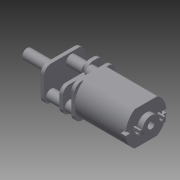
# Autodesk Inventor part: Motor
Saved by Autodesk Inventor 2015 (Build 190159000, 159)
## iProperties
Created: 2019-01-15
Part Number: Motor
Material: Типовые
Document SubType Name: Modeling
Designer: kostya
Density: 1 g/cm^3
Appearance: По умолчанию
Author: kostya
Autodesk Inventor part; units mm, degrees
ref_plane "YZ Plane" through (0, 0, 0) normal (1, 0, 0) x (0, 1, 0)
sketch "Эскиз1" plane through (0, 0, 0) normal (0, 0, 1) x (1, 0, 0)
  line L0 (-4.5, -6) -> (4.5, -6)
  line L1 (4.5, -6) -> (4.5, 6)
  line L2 (4.5, 6) -> (-4.5, 6)
  line L3 (-4.5, 6) -> (-4.5, -6)
  line L4 (-4.5, -6) -> (4.5, 6) construction
  line L5 (4.5, -6) -> (-4.5, 6) construction
  point P0 (0, 0)
  dimension "d0" = 9
  dimension "d1" = 12
  constraints: 12 end point, 2 midpoint, 2 parallel, 1 horizontal, 1 perpendicular
  measures "d0" distance of L2.end L1.end
  measures "d1" distance of L1.end L0.end
extrude "Выдавливание1" add sketch "Эскиз1" against normal blind 10
sketch "Эскиз2" plane through (4.5, -6, 0) normal (1, 0, 0) x (0, 0, -1)
  line L0 (0, 0) -> (0, 12) projected
  line L1 (0, 0) -> (10, 0) projected
  line L2 (10, 12) -> (10, 0) projected
  line L3 (0, 12) -> (10, 12) projected
  line L4 (0, 12) -> (10, 12) construction
  line L5 (5, 12) -> (5, 0) construction
  line L6 (10, 0) -> (10, 12) construction
  line L7 (10, 6) -> (0, 6) construction
  arc A0 (10, 9.3166) -> (0, 9.3166) centre (5, 6) ccw
  arc A1 (0, 2.6834) -> (10, 2.6834) centre (5, 6) ccw
  line L8 (0, 9.3166) -> (0, 2.6834)
  line L9 (0, 12) -> (0, 0) projected
  line L10 (10, 9.3166) -> (10, 2.6834)
  constraints: 8 end point, 5 point on circle, 4 midpoint, 4 point on line, 2 centre point, 1 collinear, 1 horizontal, 1 parallel
extrude "Выдавливание2" add sketch "Эскиз2" along normal blind 15 contours L0 A0 L2 A1
sketch "Эскиз3" plane through (19.5, -6, 0) normal (1, 0, 0) x (0, 0, -1)
  line L0 (0, 9.3166) -> (0, 2.6834) projected
  arc A0 (0, 2.6834) -> (10, 2.6834) centre (5, 6) ccw projected
  line L1 (10, 2.6834) -> (10, 9.3166) projected
  arc A1 (10, 9.3166) -> (0, 9.3166) centre (5, 6) ccw projected
  circle A2 centre (5, 6) radius 2.5
  circle A3 centre (5, 6) radius 1
  line L2 (5, 8.5) -> (5, 9.5) construction
  line L3 (4.25, 9.75) -> (5.75, 9.75)
  line L4 (5.75, 9.75) -> (5.75, 9.25)
  line L5 (5.75, 9.25) -> (4.25, 9.25)
  line L6 (4.25, 9.25) -> (4.25, 9.75)
  line L7 (4.25, 9.75) -> (5.75, 9.25) construction
  line L8 (5.75, 9.75) -> (4.25, 9.25) construction
  line L9 (10, 2.6834) -> (10, 9.3166) construction
  line L10 (10, 6) -> (0, 6) construction
  line L11 (4.25, 2.25) -> (5.75, 2.25)
  line L12 (5.75, 2.25) -> (5.75, 2.75)
  line L13 (5.75, 2.75) -> (4.25, 2.75)
  line L14 (4.25, 2.75) -> (4.25, 2.25)
  dimension "d6" = 5
  dimension "d7" = 2
  dimension "d9" = 1
  dimension "d10" = 1.5
  dimension "d11" = 0.5
  constraints: 24 end point, 4 symmetric about line, 3 midpoint, 2 coincident, 2 parallel, 2 perpendicular, 1 centre point, 1 horizontal, 1 vertical, 1 vertical alignment, 2 other
  measures "d7" diameter of A3
  measures "d9" distance of L2.start L2.end
  measures "d10" distance of L3.start L3.end
  measures "d11" distance of L3.end L4.end
extrude "Выдавливание3" add sketch "Эскиз3" along normal blind 1.5 contours A2
extrude "Выдавливание4" add sketch "Эскиз3" along normal blind 2 contours L3 L4 L5 L6 | L14 L13 L12 L11
sketch "Эскиз4" plane through (19.5, 3.75, -4.25) normal (0, 1, 0) x (1, 0, 0)
  line L0 (0, 0) -> (0, 1.5) projected
  line L1 (0, 0) -> (2, 0) projected
  line L2 (2, 1.5) -> (2, 0) projected
  line L3 (0, 1.5) -> (2, 1.5) projected
  circle A0 centre (1, 0.75) radius 0.65
  point P0 (-19.5, -4.25)
  dimension "d16" = 1.3
  constraints: 1 centre point
  measures "d16" diameter of A0
extrude "Выдавливание5" cut sketch "Эскиз4" against normal blind 1 contours A0
ref_plane "РабПлоскость1" through (19.5, 0, -4.25) normal (0, 1, 0) x (1, 0, 0)
mirror "Зеркальное отражение1" about plane through (19.5, 0, -4.25) normal (0, 1, 0) of "Выдавливание5"
sketch "Эскиз5" plane through (19.5, -6, 0) normal (1, 0, 0) x (0, 0, -1)
  line L0 (5.75, 9.75) -> (5.75, 9.25) projected
  line L1 (5.75, 9.25) -> (4.25, 9.25) projected
  line L2 (4.25, 9.25) -> (4.25, 9.75) projected
  line L3 (4.25, 9.75) -> (5.75, 9.75) projected
  line L4 (4.25, 2.25) -> (4.25, 2.75) projected
  line L5 (4.25, 2.75) -> (5.75, 2.75) projected
  line L6 (5.75, 2.75) -> (5.75, 2.25) projected
  line L7 (5.75, 2.25) -> (4.25, 2.25) projected
  line L8 (0, 9.3166) -> (0, 2.6834) projected
  arc A0 (0, 2.6834) -> (10, 2.6834) centre (5, 6) ccw projected
  line L9 (10, 2.6834) -> (10, 9.3166) projected
  arc A1 (10, 9.3166) -> (0, 9.3166) centre (5, 6) ccw projected
  circle A2 centre (5, 6) radius 2.5 projected
  line L10 (5, 2.25) -> (5, 1.25) construction
  line L11 (5.5, 1.25) -> (5, 1.25) construction
  line L12 (5, 1.25) -> (4.5, 1.25) construction
  line L13 (4.5, 1.25) -> (5.5, 1.25)
  line L14 (5.5, 1.25) -> (5.5, -0.0734)
  line L15 (5.5, -0.0734) -> (4.5, -0.0734)
  line L16 (4.5, -0.0734) -> (4.5, 1.25)
  line L17 (5, 6) -> (10, 6) construction
  line L18 (10, 2.6834) -> (10, 9.3166) construction
  line L19 (5, 9.75) -> (5, 10.75) construction
  line L20 (5.5, 10.75) -> (5, 10.75) construction
  line L21 (4.5, 10.75) -> (5.5, 10.75)
  line L22 (5.5, 10.75) -> (5.5, 12.0734)
  line L23 (5.5, 12.0734) -> (4.5, 12.0734)
  line L24 (4.5, 12.0734) -> (4.5, 10.75)
  point P0 (0, 6)
  dimension "d19" = 1
  dimension "d20" = 0.5
  constraints: 28 end point, 7 symmetric about line, 2 horizontal, 2 midpoint, 2 parallel, 2 point on line, 1 perpendicular, 1 vertical
  measures "d19" distance of L10.start L10.end
  measures "d20" distance of L10.end L12.end
extrude "Выдавливание6" cut sketch "Эскиз5" against normal blind 1.5 contours L24 L23 L22 A1 | A1 L22 L21 L24 | L16 L13 L14 A0 | A0 L14 L15 L16
sketch "Эскиз6" plane through (-4.5, -6, 0) normal (0, -1, 0) x (1, 0, 0)
  line L0 (0, 0) -> (9, 0) projected
  line L1 (0, 0) -> (0, -10) projected
  line L2 (9, -10) -> (0, -10) projected
  line L3 (9, -5) -> (9, -10) projected
  line L4 (9, 0) -> (9, -5) projected
  line L5 (9, 0) -> (8, 0)
  line L6 (8, 0) -> (8, -10)
  line L7 (8, -10) -> (9, -10)
  line L8 (9, -10) -> (9, 0)
  point P0 (4.5, 0)
  dimension "d23" = 1
  constraints: 8 end point, 2 parallel, 1 horizontal, 1 perpendicular, 1 point on line
  measures "d23" distance of L7.end L6.end
extrude "Выдавливание7" cut sketch "Эскиз6" against normal up to next contours L0 L6 L2 L1
sketch "Эскиз7" plane through (3.5, -6, -10) normal (-1, 0, 0) x (0, 0, 1)
  line L0 (0, 12) -> (10, 12) projected
  line L1 (0, 0) -> (0, 12) projected
  line L2 (10, 0) -> (0, 0) projected
  line L3 (10, 12) -> (10, 0) projected
  line L4 (0, 0) -> (1, 0) construction
  line L5 (1, 0) -> (1, 1) construction
  line L6 (1, 1) -> (0, 1) construction
  line L7 (0, 1) -> (0, 0) construction
  line L8 (1, 1) -> (3.1213, 3.1213) construction
  line L9 (1, 1) -> (4, 1) construction
  circle A0 centre (2.0607, 2.0607) radius 1.5
  point P0 (10, 6)
  dimension "d26" = 1
  dimension "d27" = 1
  dimension "d28" = 3
  dimension "d29" = 45
  constraints: 12 end point, 2 horizontal, 2 parallel, 1 equal length, 1 midpoint, 1 perpendicular, 3 other
  measures "d26" distance of L6.end L5.end
  measures "d27" distance of L5.end L4.end
  measures "d28" distance of L5.end L8.end
  measures "d29" angle of L9 L8
extrude "Выдавливание8" add sketch "Эскиз7" along normal blind 2.5 contours A0
sketch "Эскиз8" plane through (4.5, -6, -10) normal (0, -1, 0) x (1, 0, 0)
  line L0 (-3.5, 3.5607) -> (-3.5, 0.5607) projected
  line L1 (-1, 0.5607) -> (-1, 3.5607) projected
  line L2 (-1, 10) -> (-1, 0) construction
  line L3 (0, 0) -> (-1, 0) construction
  line L4 (0, 5) -> (0, 0) construction
  line L5 (0, 10) -> (0, 5) construction
  line L6 (-1, 10) -> (0, 10) construction
  line L7 (0, 0) -> (-4.7525, 0) construction
  line L8 (-3.5, 0.5607) -> (-3.5, 0) construction
  line L9 (-3.5, 0) -> (-4.5, 0)
  line L10 (-4.5, 0) -> (-4.5, 10)
  line L11 (-4.5, 10) -> (-3.5, 10)
  line L12 (-3.5, 10) -> (-3.5, 0)
  dimension "d32" = 1
  constraints: 12 end point, 2 horizontal, 2 parallel, 2 perpendicular, 1 point on line
  measures "d32" distance of L10.end L11.end
extrude "Выдавливание9" add sketch "Эскиз8" against normal up to surface (12 mm away)
sketch "Эскиз9" plane through (0, -6, -10) normal (-1, 0, 0) x (0, 0, 1)
  line L0 (10, 12) -> (0, 12) projected
  line L1 (0, 0) -> (0, 12) projected
  line L2 (10, 0) -> (0, 0) projected
  line L3 (10, 0) -> (10, 12) projected
  line L4 (10, 12) -> (10, 7) construction
  line L5 (10, 12) -> (10, 0) construction
  line L6 (0, 0) -> (7.5, 0) construction
  line L7 (10, 0) -> (0, 0) construction
  line L8 (10, 7) -> (7.5, 7)
  line L9 (7.5, 7) -> (7.5, 0)
  line L10 (7.5, 0) -> (10, 0)
  line L11 (10, 0) -> (10, 7)
  point P0 (10, 6)
  dimension "d35" = 5
  dimension "d36" = 7.5
  constraints: 12 end point, 2 parallel, 2 point on line, 1 horizontal, 1 perpendicular
  measures "d35" distance of L0.start L4.end
  measures "d36" distance of L1.start L6.end
extrude "Выдавливание10" cut sketch "Эскиз9" against normal blind 2.5 contours L3 L2 L9 L8
sketch "Эскиз10" plane through (0, -6, -10) normal (-1, 0, 0) x (0, 0, 1)
  line L0 (7.5, 7) -> (10, 7) projected
  line L1 (10, 7) -> (10, 12) projected
  line L2 (10, 12) -> (0, 12) projected
  line L3 (0, 0) -> (0, 12) projected
  line L4 (7.5, 0) -> (0, 0) projected
  line L5 (7.5, 0) -> (7.5, 7) projected
  circle A0 centre (2.0607, 2.0607) radius 1.5 projected
  point P0 (10, 6)
extrude "Выдавливание11" add sketch "Эскиз10" along normal blind 4.5 contours A0
sketch "Эскиз11" plane through (4.5, -6, -10) normal (0, -1, 0) x (1, 0, 0)
  line L0 (-3.5, 7.5) -> (-4.5, 7.5) projected
  line L1 (-4.5, 7.5) -> (-4.5, 0) projected
  line L2 (-4.5, 0) -> (-3.5, 0) projected
  line L3 (-3.5, 0) -> (-3.5, 7.5) projected
  line L4 (-3.5, 10) -> (-3.5, 7.5) projected
  line L5 (-4.5, 10) -> (-3.5, 10) projected
  line L6 (-4.5, 7.5) -> (-4.5, 10) projected
  line L7 (-4.5, 7.5) -> (-3.5, 7.5) projected
  line L8 (-1, 10) -> (-1, 0) projected
  line L9 (0, 0) -> (-1, 0) projected
  line L10 (0, 5) -> (0, 0) projected
  line L11 (0, 10) -> (0, 5) projected
  line L12 (-1, 10) -> (0, 10) projected
  line L13 (-9, 3.5607) -> (-9, 0.5607) projected
  line L14 (-4.5, 0.5607) -> (-4.5, 3.5607) projected
  line L15 (-9, 0.5607) -> (-9, 0) construction
  line L16 (-9, 0) -> (0, 0) construction
  line L17 (-9, 0) -> (-10, 0)
  line L18 (-10, 0) -> (-10, 10)
  line L19 (-10, 10) -> (-9, 10)
  line L20 (-9, 10) -> (-9, 0)
  dimension "d41" = 1
  constraints: 12 end point, 2 parallel, 2 perpendicular, 1 horizontal, 1 vertical
  measures "d41" distance of L18.end L19.end
extrude "Выдавливание12" add sketch "Эскиз11" against normal up to surface (12 mm away) contours L13 L20 L17 L18 L19
ref_plane "РабПлоскость3" through (4.5, -6, 0) normal (0, -0.7071068, -0.7071068) x (1, 0, 0)
mirror "Зеркальное отражение2" about plane through (4.5, -6, 0) normal (0, -0.7071068, -0.7071068) of "Выдавливание11", "Выдавливание8"
fillet "Сопряжение1" radius 2 13 edges at (-5, -6, 0) (0.5, -6, -2.5) (4, -6, 0) (-5, 6, 0) (0.5, 6, 0) (4, 6, 0) (0.5, 1, 0) (0.5, -6, -10) (4, -6, -10) (-5, -6, -10) (-5, 6, -10) (0.5, 6, -10) (4, 6, -10)
sketch "Эскиз12" plane through (-5.5, -6, -8) normal (-1, 0, 0) x (0, 0, 1)
  arc A0 (0, 12) -> (-2, 10) centre (0, 10) ccw projected
  line L0 (-2, 2) -> (-2, 10) projected
  arc A1 (-2, 2) -> (0, 0) centre (0, 2) ccw projected
  line L1 (0, 0) -> (6, 0) projected
  arc A2 (6, 0) -> (8, 2) centre (6, 2) ccw projected
  line L2 (8, 2) -> (8, 10) projected
  arc A3 (8, 10) -> (6, 12) centre (6, 10) ccw projected
  line L3 (6, 12) -> (0, 12) projected
  line L4 (8, 6) -> (-2, 6) construction
  line L5 (-2, 2) -> (-2, 10) construction
  line L6 (0, 12) -> (6, 12) construction
  line L7 (3, 12) -> (3, 0) construction
  line L8 (0, 0) -> (6, 0) construction
  arc A4 (2, 4.882) -> (2, 7.118) centre (3, 6) ccw
  line L9 (4.5, 6) -> (2, 6) construction
  line L10 (2, 6) -> (2, 4.882) construction
  line L11 (2, 7.118) -> (2, 4.882)
  dimension "d45" = 3
  dimension "d46" = 2.5
  constraints: 10 end point, 4 midpoint, 3 point on circle, 2 point on line, 1 centre point, 1 collinear, 1 perpendicular
  measures "d45" diameter of A4
  measures "d46" distance of L9.start L9.end
extrude "Выдавливание13" add sketch "Эскиз12" along normal blind 10 contours L11 A4
sketch "Эскиз13" plane through (-5.5, -6, -8) normal (-1, 0, 0) x (0, 0, 1)
  arc A0 (2, 4.882) -> (2, 7.118) centre (3, 6) ccw projected
  line L0 (2, 7.118) -> (2, 4.882) projected
  circle A1 centre (3, 6) radius 2
  point P0 (8, 6)
  dimension "d49" = 4
  constraints: 1 centre point, 1 coincident
  measures "d49" diameter of A1
extrude "Выдавливание14" add sketch "Эскиз13" along normal blind 1
